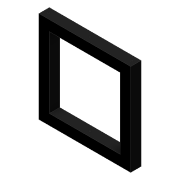
# Autodesk Inventor part: sambung kotak
Saved by Autodesk Inventor 2018 (Build 220112000, 112)
## iProperties
Created: 2019-12-19
Part Number: sambung kotak
Material: Generic
Document SubType Name: Modeling
Designer: Ibnu
Density: 1 g/cm^3
Appearance: Default
Mass: 484.036 g
Surface Area: 825.616 cm^2
Volume: 484.036 cm^3
Author: Ibnu
Autodesk Inventor part; units mm, degrees
ref_plane "YZ Plane" through (0, 0, 0) normal (1, 0, 0) x (0, 1, 0)
ref_plane "XZ Plane" through (0, 0, 0) normal (0, 1, 0) x (-1, 0, 0)
sketch "Sketch1" plane through (0, 0, 0) normal (0, 1, 0) x (-1, 0, 0)
  line L0 (0, 170) -> (0, 0)
  line L1 (-195, -25) -> (-25, -25)
  line L2 (-220, 0) -> (-220, 170)
  line L3 (-25, 195) -> (-195, 195)
  line L4 (-25, 195) -> (0, 195)
  line L5 (0, 195) -> (0, 170)
  line L6 (0, 0) -> (0, -25)
  line L7 (0, -25) -> (-25, -25)
  line L8 (-195, -25) -> (-220, -25)
  line L9 (-220, -25) -> (-220, 0)
  line L10 (-220, 170) -> (-220, 195)
  line L11 (-195, 195) -> (-220, 195)
  line L12 (-25, 170) -> (-195, 170)
  line L13 (-195, 170) -> (-195, 0)
  line L14 (-195, 0) -> (-25, 0)
  line L15 (-25, 0) -> (-25, 170)
  line L16 (-25, 170) -> (-195, 0) construction
  line L17 (-195, 170) -> (-25, 0) construction
  point P0 (-110, 85)
  dimension "d2" = 170
  dimension "d5" = 170
  dimension "d7" = 170
  dimension "d8" = 170
  constraints: 36 end point, 5 perpendicular, 4 point on line, 2 horizontal, 2 midpoint, 2 parallel
  measures "d2" distance of L1.end L1.start
  measures "d5" distance of L2.start L2.end
  measures "d7" distance of L14.end L13.end
  measures "d8" distance of L13.end L12.end
extrude "Extrusion1" add sketch "Sketch1" along normal blind 25
ref_plane "Work Plane1" through (0, 0, -20) normal (0, 0, 1) x (1, 0, 0)
sketch "Sketch2" plane through (0, 0, -20) normal (0, 0, 1) x (1, 0, 0)
  line L0 (0, 0) -> (0, 25) projected
  circle A0 centre (10, 12.5) radius 1.5
  line L1 (220, 0) -> (220, 25) projected
  circle A1 centre (210, 12.5) radius 1.5
  constraints: 2 centre point
extrude "Extrusion2" cut sketch "Sketch2" along normal through all both and the other way through all
sketch "Sketch3" plane through (0, 0, 195) normal (0, 0, 1) x (1, 0, 0)
  line L0 (195, 25) -> (25, 25) projected
  circle A0 centre (110, 12.5) radius 1.5
  constraints: 1 centre point
hole "Hole1" at (110, 12.5, 195) direction (0, 0, -1) diameter 3 end through all
body "Solid1"
